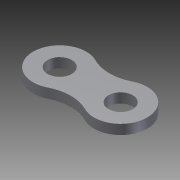
# Autodesk Inventor part: Concha2
Saved by Autodesk Inventor 2011 (Build 150239000, 239)
## iProperties
Created: 2011-08-31
Part Number: Concha2
Document SubType Name: Modeling
Designer: Luis
Density: 1 g/cm^3
Author: Luis
Autodesk Inventor part; units mm, degrees
ref_plane "YZ Plane" through (0, 0, 0) normal (1, 0, 0) x (0, 1, 0)
ref_plane "XZ Plane" through (0, 0, 0) normal (0, 1, 0) x (-1, 0, 0)
ref_plane "XY Plane" through (0, 0, 0) normal (0, 0, 1) x (1, 0, 0)
sketch "Sketch1" plane through (0, 0, 0) normal (0, 0, 1) x (1, 0, 0)
  line L0 (-6.3, 0) -> (6.3, 0) construction
  circle A0 centre (-6.3, 0) radius 2.5
  circle A1 centre (6.3, 0) radius 2.5
  arc A2 (-3.7701, 4.8836) -> (-3.7701, -4.8836) centre (-6.3, 0) ccw
  arc A3 (3.7701, -4.8836) -> (3.7701, 4.8836) centre (6.3, 0) ccw
  line L1 (0, 0) -> (0, 4) construction
  line L2 (0, 0) -> (0, -4) construction
  arc A4 (-3.7701, 4.8836) -> (3.7701, 4.8836) centre (0, 12.4848) ccw
  arc A5 (3.7701, -4.8836) -> (-3.7701, -4.8836) centre (0, -12.4848) ccw
  dimension "d0" = 12.6
  dimension "d1" = 5
  dimension "d2" = 5
  dimension "d3" = 11
  dimension "d4" = 11
  dimension "d5" = 4
  dimension "d6" = 4
  constraints: 9 point on circle, 6 centre point, 6 end point, 5 coincident, 3 symmetric about line, 1 collinear, 1 horizontal, 1 midpoint, 1 perpendicular, 1 other
  measures "d0" distance of L0.start L0.end
  measures "d1" diameter of A0
  measures "d2" diameter of A1
  measures "d3" diameter of A2
  measures "d4" diameter of A3
  measures "d5" distance of L1.start L1.end
  measures "d6" distance of L1.start L2.end
extrude "Extrusion1" add sketch "Sketch1" along normal blind 2
body "Solid1"
